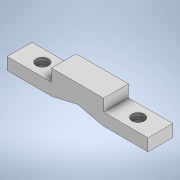
# Autodesk Inventor part: syringe holder
Saved by Autodesk Inventor 2022 (Build 260153000, 153)
## iProperties
Created: 2022-04-24
Part Number: syringe holder
Material: Generic
Document SubType Name: Modeling
Designer: vitalii
Density: 1 g/cm^3
Appearance: Default
Author: vitalii
Autodesk Inventor part; units mm, degrees
ref_plane "YZ Plane" through (0, 0, 0) normal (1, 0, 0) x (0, 1, 0)
ref_plane "XZ Plane" through (0, 0, 0) normal (0, 1, 0) x (-1, 0, 0)
ref_plane "XY Plane" through (0, 0, 0) normal (0, 0, 1) x (1, 0, 0)
sketch "Sketch1" plane through (0, 0, 0) normal (0, 0, 1) x (1, 0, 0)
  line L0 (-14.4256, 5.5876) -> (8.1894, 5.5876)
  line L1 (8.1894, 5.5876) -> (8.1894, 11.7876)
  line L2 (8.1894, 11.7876) -> (34.7894, 11.7876)
  line L3 (34.7894, 11.7876) -> (34.7894, 5.5876)
  line L4 (34.7894, 5.5876) -> (57.4044, 5.5876)
  line L5 (57.4044, 5.5876) -> (57.4044, -0.6124)
  line L6 (57.4044, -0.6124) -> (34.4294, -0.6124)
  line L7 (-14.4256, 5.5876) -> (-14.4256, -0.6124)
  line L8 (-14.4256, -0.6124) -> (8.5494, -0.6124)
  line L9 (21.4894, 2.3876) -> (8.5494, -0.6124)
  line L10 (21.4894, 2.3876) -> (34.4294, -0.6124)
  point P0 (0, 0)
  dimension "d0" = 22.615
  dimension "d1" = 6.2
  dimension "d2" = 26.6
  dimension "d3" = 22.615
  dimension "d4" = 6.2
  dimension "d5" = 22.975
  dimension "d9" = 22.975
  constraints: 22 end point, 6 perpendicular, 2 point on line, 1 horizontal, 1 vertical
  measures "d0" distance of L0.start L0.end
  measures "d1" distance of L0.end L1.end
  measures "d2" distance of L1.end L2.end
  measures "d3" distance of L3.end L4.end
  measures "d4" distance of L4.end L5.end
  measures "d5" distance of L5.end L6.end
  measures "d9" distance of L7.end L8.end
extrude "Extrusion1" add sketch "Sketch1" against normal blind 12.64
sketch "Sketch2" plane through (-14.4256, 5.5876, 0) normal (0, 1, 0) x (1, 0, 0)
  circle A0 centre (11.488, 6.46) radius 3.175
  circle A1 centre (60.342, 6.46) radius 3.175
  line L0 (0, 0) -> (0, 12.64) projected
  line L1 (0, 12.64) -> (22.615, 12.64) projected
  line L2 (49.215, 12.64) -> (71.83, 12.64) projected
  line L3 (71.83, 0) -> (71.83, 12.64) projected
  point P0 (14.4256, 0)
  dimension "d14" = 11.488
  dimension "d15" = 6.18
  dimension "d16" = 6.35
  dimension "d17" = 6.18
  dimension "d18" = 11.488
  dimension "d19" = 6.35
  constraints: 2 centre point
  measures "d14" distance from line of L0 A0.centre
  measures "d15" distance from line of L1 A0.centre
  measures "d16" diameter of A0
  measures "d17" distance from line of L2 A1.centre
  measures "d18" distance from line of L3 A1.centre
  measures "d19" diameter of A1
extrude "Extrusion2" cut sketch "Sketch2" against normal blind 12.64
thread "Thread1" size "1/4-20 UNC" class "2B" standard "ANSI Unified Screw Threads" full length
thread "Thread2" size "1/4-20 UNC" class "2B" standard "ANSI Unified Screw Threads" full length
body "Solid1"
